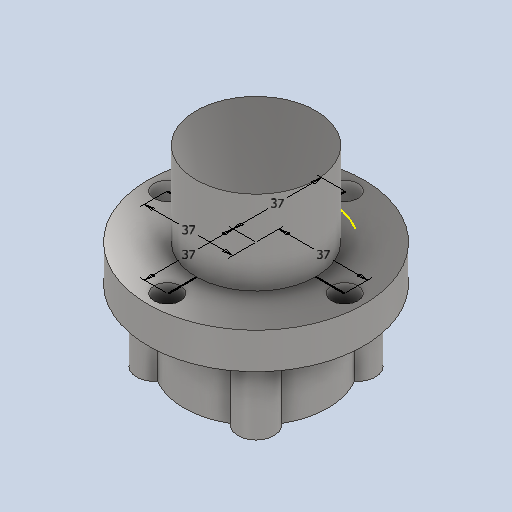
# Autodesk Inventor part: КреплениеБарабана
Saved by Autodesk Inventor 2024.2 (Build 282272000, 272)
## iProperties
Created: 2025-03-01
Part Number: КреплениеБарабана
Material: Сталь, литейная
Document SubType Name: Modeling
Designer: Timofey
Density: 7.85 g/cm^3
Appearance: С умеренной полировкой
Mass: 2001.3 g
Surface Area: 306.52 cm^2
Volume: 254.942 cm^3
Author: Timofey
Autodesk Inventor part; units mm, degrees
ref_plane "YZ Plane" through (0, 0, 0) normal (1, 0, 0) x (0, 1, 0)
ref_plane "XZ Plane" through (0, 0, 0) normal (0, 1, 0) x (-1, 0, 0)
ref_plane "XY Plane" through (0, 0, 0) normal (0, 0, 1) x (1, 0, 0)
sketch "Эскиз1" plane through (0, 0, 0) normal (0, 1, 0) x (-1, 0, 0)
  circle A0 centre (0, 0) radius 45
  dimension "d0" = 90
  constraints: 1 centre point, 1 coincident
  measures "d0" diameter of A0
extrude "Выдавливание1" add sketch "Эскиз1" along normal blind 15
sketch "Эскиз3" plane through (0, 0, 0) normal (0, -1, 0) x (1, 0, 0)
  circle A0 centre (0, 0) radius 30
  line L0 (-15.9099, 15.9099) -> (-21.2132, 21.2132)
  line L1 (0, 0) -> (30, 0) construction
  line L2 (-15.9099, -15.9099) -> (-21.2132, -21.2132)
  line L3 (0, 0) -> (30, 0) construction
  line L4 (15.9099, -15.9099) -> (21.2132, -21.2132)
  line L5 (0, 0) -> (30, 0) construction
  line L6 (15.9099, 15.9099) -> (21.2132, 21.2132)
  line L7 (0, 0) -> (30, 0) construction
  arc A1 (-25.812, -15.2886) -> (-15.2886, -25.812) centre (-21.2132, -21.2132) ccw
  arc A2 (-15.2886, 25.812) -> (-25.812, 15.2886) centre (-21.2132, 21.2132) ccw
  arc A3 (25.812, 15.2886) -> (15.2886, 25.812) centre (21.2132, 21.2132) ccw
  arc A4 (15.2886, -25.812) -> (25.812, -15.2886) centre (21.2132, -21.2132) ccw
  dimension "d26" = 60
  dimension "d27" = 30
  dimension "d28" = 135
  dimension "d29" = 30
  dimension "d30" = 135
  dimension "d31" = 30
  dimension "d32" = 45
  dimension "d33" = 30
  dimension "d34" = 45
  dimension "d35" = 15
  dimension "d36" = 15
  dimension "d37" = 15
  dimension "d38" = 15
  constraints: 16 end point, 9 point on circle, 5 coincident, 4 centre point, 4 horizontal, 10 other
  measures "d27" distance of L1.start L0.end
  measures "d28" angle of L1 L0
  measures "d29" distance of L1.start L2.end
  measures "d30" angle of L2 L3
  measures "d31" distance of L1.start L4.end
  measures "d32" angle of L4 L5
  measures "d33" distance of L1.start L6.end
  measures "d34" angle of L7 L6
  measures "d35" diameter of A1
  measures "d36" diameter of A2
  measures "d37" diameter of A3
  measures "d38" diameter of A4
extrude "Выдавливание2" add sketch "Эскиз3" along normal blind 30
sketch "Эскиз4" plane through (0, 15, 0) normal (0, 1, 0) x (1, 0, 0)
  circle A0 centre (0, 0) radius 25
  dimension "d41" = 50
  constraints: 1 centre point, 1 coincident
  measures "d41" diameter of A0
extrude "Выдавливание3" add sketch "Эскиз4" along normal blind 35
sketch "Эскиз5" plane through (0, 15, 0) normal (0, 1, 0) x (1, 0, 0)
  line L0 (0, 0) -> (0, -37)
  arc A0 (15.2886, 25.812) -> (-15.2886, 25.812) centre (0, 0) ccw projected
  line L1 (0, 0) -> (37, 0)
  line L2 (0, 0) -> (0, 37)
  line L3 (0, 0) -> (-37, 0)
  dimension "d44" = 37
  dimension "d45" = 37
  dimension "d46" = 37
  dimension "d47" = 37
  constraints: 8 end point, 2 horizontal, 2 vertical
  measures "d44" distance of L0.start L0.end
  measures "d45" distance of L1.start L1.end
  measures "d46" distance of L1.start L2.end
  measures "d47" distance of L1.start L3.end
sketch "Эскиз6" plane through (0, 15, 0) normal (0, 1, 0) x (1, 0, 0)
  point P0 (37, 0)
  point P1 (0, -37)
  point P2 (-37, 0)
  point P3 (0, 37)
hole "Отверстие2" at (37, 15, 0) at (0, 15, 37) at (-37, 15, 0) at (0, 15, -37) direction (0, -1, 0) diameter 11 end through all
